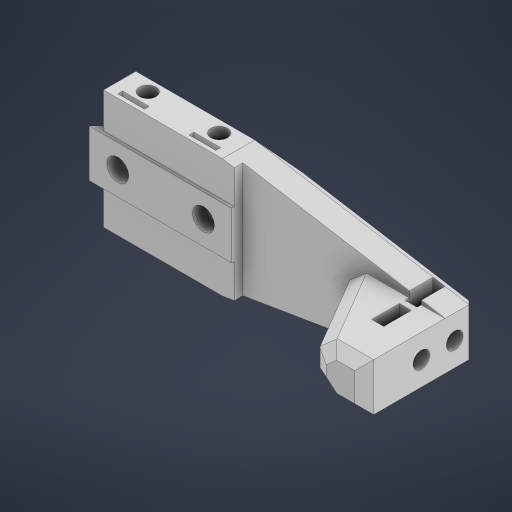
# Autodesk Inventor part: Lupfer oben
Saved by Autodesk Inventor 2024.2 (Build 282272000, 272)
## iProperties
Created: 2023-12-02
Part Number: Lupfer oben
Material: Generisch
Document SubType Name: Modeling
Designer: jacob
Density: 1 g/cm^3
Appearance: Vorgabe
Author: jacob
Autodesk Inventor part; units mm, degrees
ref_plane "YZ Plane" through (0, 0, 0) normal (1, 0, 0) x (0, 1, 0)
ref_plane "XZ Plane" through (0, 0, 0) normal (0, 1, 0) x (-1, 0, 0)
ref_plane "XY Plane" through (0, 0, 0) normal (0, 0, 1) x (1, 0, 0)
sketch "Skizze1" plane through (0, 0, 0) normal (0, 0, 1) x (1, 0, 0)
  line L0 (0, 0) -> (0, -12.5)
  line L1 (0, -12.5) -> (25, -12.5)
  line L2 (25, -12.5) -> (25, -5)
  line L3 (25, -5) -> (70, -5)
  line L4 (70, -5) -> (70, 0)
  line L5 (0, 0) -> (70, 0)
  line L6 (25, -12.5) -> (70, -5)
  dimension "d0" = 25
  dimension "d1" = 12.5
  dimension "d3" = 5
  dimension "d31" = 70
  constraints: 14 end point, 4 perpendicular, 1 horizontal, 1 horizontal alignment, 1 vertical
  measures "d0" distance of L0.end L1.end
  measures "d1" distance of L0.start L0.end
  measures "d3" distance between parallel lines of L5 L3
  measures "d31" distance of L4.end L0.start
extrude "Extrusion1" add sketch "Skizze1" along normal blind 5
sketch "Skizze2" plane through (0, 0, 5) normal (0, 0, 1) x (1, 0, 0)
  line L0 (70, 0) -> (0, 0) projected
  line L1 (0, 0) -> (0, -12.5) projected
  point P0 (3.5, 0)
  point P1 (0, 0)
  point P2 (21.5, 0)
  dimension "d7" = 3.5
  dimension "d84" = 18
  constraints: 1 horizontal alignment, 1 point on line
  measures "d7" distance of L0.end point (3.5, 0)
  measures "d84" distance of point (3.5, 0) point (21.5, 0)
hole "Bohrung1" at (3.5, 0, 5) at (21.5, 0, 5) direction (0, 0, -1) diameter 3.5 end through all
sketch "Skizze3" plane through (0, -12.5, 0) normal (0, -1, 0) x (1, 0, 0)
  line L0 (0, 0) -> (0, 5) projected
  line L1 (0, 2.5) -> (5, 2.5) construction
  line L2 (20, 2.5) -> (25, 2.5) construction
  point P0 (25, 0)
  dimension "d15" = 15
  constraints: 4 end point, 4 horizontal alignment, 3 midpoint, 2 horizontal, 1 collinear, 1 vertical alignment
  measures "d15" distance of L1.end L2.start
sketch "Skizze4" plane through (0, 0, 5) normal (0, 0, 1) x (1, 0, 0)
  line L0 (2.2, -5) -> (7.8, -5)
  line L1 (7.8, -5) -> (7.8, -7.5)
  line L2 (7.8, -7.5) -> (2.2, -7.5)
  line L3 (2.2, -7.5) -> (2.2, -5)
  line L4 (17.2, -5) -> (22.8, -5)
  line L5 (22.8, -5) -> (22.8, -7.5)
  line L6 (22.8, -7.5) -> (17.2, -7.5)
  line L7 (17.2, -7.5) -> (17.2, -5)
  line L8 (5, -5) -> (0, -5) construction
  line L9 (20, -5) -> (25, -5) construction
  line L10 (0, -12.5) -> (25, -12.5) projected
  line L11 (0, 0) -> (0, -12.5) projected
  line L12 (25, -12.5) -> (25, 0)
  line L13 (70, 0) -> (23.25, 0) projected
  dimension "d17" = 5.6
  dimension "d18" = 2.5
  dimension "d20" = 15
  dimension "d21" = 5
  constraints: 22 end point, 5 point on line, 4 parallel, 3 equal length, 3 horizontal, 3 perpendicular, 2 midpoint, 1 vertical
  measures "d17" distance of L0.start L0.end
  measures "d18" distance of L0.end L1.end
  measures "d20" distance of L9.start L8.start
  measures "d21" distance from line of L10 L5.end
extrude "Extrusion2" cut sketch "Skizze4" against normal blind 5
hole "Bohrung2" at (5, -12.5, 2.5) at (20, -12.5, 2.5) direction (0, 1, 0) diameter 3.5 depth 9 tip angle 90
mirror "Spiegeln2" about plane through (70, 0, 0) normal (0, 1, 0) of "Extrusion1", "Bohrung1", "Extrusion2", "Bohrung2"
sketch "Skizze13" plane through (0, 0, 0) normal (0, 1, 0) x (-1, 0, 0)
  line L0 (-70, 0) -> (-70, 5) projected
  line L1 (-70, 0) -> (-70, -5)
  line L2 (-70, -5) -> (0, -5)
  line L3 (0, -5) -> (0, 0)
  line L4 (0, 0) -> (-70, 0)
  dimension "d80" = 5
  dimension "d116" = 90
  constraints: 8 end point, 3 perpendicular
  measures "d80" distance of L2.end L3.end
  measures "d116" angle of L4 L1
extrude "Extrusion6" add sketch "Skizze13" along normal mid plane 10
sketch "Skizze14" plane through (21.5, 0, 0) normal (0, 0, 1) x (1, 0, 0)
  circle A0 centre (0, 0) radius 1.75 projected
  circle A1 centre (-18, 0) radius 1.75 projected
  point P0 (-21.5, 0)
  point P1 (-4, 0)
  constraints: 2 coincident
hole "Bohrung7" at (21.5, 0, 0) at (3.5, 0, 0) direction (0, 0, -1) diameter 6 end through all
sketch "Skizze15" plane through (0, 0, 0) normal (0, 1, 0) x (-1, 0, 0)
  line L0 (-70, 0) -> (-70, 5) projected
  line L1 (-70, 5) -> (-70, 22)
  line L2 (-70, 22) -> (-60, 22)
  line L3 (-60, 22) -> (-50, 5)
  line L4 (-50, 5) -> (-70, 5)
  point P0 (0, 0)
  dimension "d92" = 20
  dimension "d93" = 10
  dimension "d94" = 17
  constraints: 8 end point, 2 perpendicular, 1 vertical
  measures "d92" distance of L3.end L0.end
  measures "d93" distance of L1.end L2.end
  measures "d94" distance of L0.end L1.end
extrude "Extrusion7" add sketch "Skizze15" along normal mid plane 10
sketch "Skizze16" plane through (0, -5, 0) normal (0, -1, 0) x (1, 0, 0)
  point P0 (0, 0)
sketch "Skizze17" plane through (0, -5, 0) normal (0, -1, 0) x (1, 0, 0)
  line L0 (62.5, 0.1) -> (62.5, 5.9)
  line L1 (62.5, 5.9) -> (65, 5.9)
  line L2 (65, 5.9) -> (65, 0.1)
  line L3 (65, 7.1) -> (62.5, 7.1)
  line L4 (62.5, 7.1) -> (62.5, 12.9)
  line L5 (62.5, 12.9) -> (65, 12.9)
  line L6 (65, 12.9) -> (65, 7.1)
  line L7 (70, 5) -> (70, 22) projected
  line L8 (70, 22) -> (60, 22) construction
  line L9 (62.5, 0.1) -> (65, 0.1)
  line L10 (70, 0) -> (22.8, 0) construction
  point P0 (0, 0)
  point P1 (63.75, 5.9)
  point P2 (63.75, 7.1)
  point P3 (62.5, 10)
  point P4 (62.5, 3)
  point P5 (23, 0)
  dimension "d97" = 5.8
  dimension "d98" = 2.5
  dimension "d99" = 5
  dimension "d111" = 7
  dimension "d115" = 12
  constraints: 16 end point, 4 midpoint, 3 horizontal, 3 parallel, 2 equal length, 1 perpendicular, 1 vertical alignment
  measures "d97" distance of L0.start L0.end
  measures "d98" distance of L2.end L0.start
  measures "d99" distance between parallel lines of L7 L2
  measures "d111" distance of point (62.5, 10) point (62.5, 3)
  measures "d115" distance from line of L8 point (62.5, 10)
extrude "Extrusion8" cut sketch "Skizze17" along normal through all both and the other way through all
sketch "Skizze18" plane through (70, -5, 0) normal (1, 0, 0) x (0, 0, -1)
  line L0 (-22, 0) -> (-22, 10) construction
  line L1 (0, 10) -> (0, 0)
  line L2 (0, 6.75) -> (0, 3.25) projected
  point P0 (-10, 5)
  point P1 (-3, 5)
  point P2 (0, 5)
  point P3 (0, 5)
  dimension "d109" = 7
  dimension "d160" = 12
  constraints: 2 end point, 2 horizontal alignment, 2 midpoint, 1 vertical
  measures "d109" distance of point (-3, 5) point (-10, 5)
  measures "d160" distance from line of L0 point (-10, 5)
hole "Bohrung8" at (70, 0, 3) at (70, 0, 10) direction (-1, 0, 0) diameter 3.5 depth 12 tip angle 90
sketch "Skizze19" plane through (0, 0, 0) normal (0, 0, -1) x (-1, 0, 0)
  line L0 (-25, -12.5) -> (-70, -5) projected
  line L1 (-25, -12.5) -> (-25, -5)
  line L2 (0, -5) -> (-70, -5) projected
  line L3 (-22.8, -5) -> (-70, -5) projected
  line L4 (-25, -5) -> (-70, -5)
  line L5 (-70, -5) -> (-62.5, -6.25)
  point P0 (0, 0)
  constraints: 6 end point, 1 collinear, 1 horizontal, 1 point on line, 1 vertical
extrude "Extrusion9" add sketch "Skizze19" along normal up to surface (5 mm away)
mirror "Spiegeln3" about plane through (0, 0, 0) normal (0, 1, 0) of "Extrusion9"
chamfer "Fasen3" distance 5 angle 45 1 edges at (70, 0, -5)
chamfer "Fasen4" distance 5 angle 45 4 edges at (25, -8.75, -5) (45, -9.1667, -5) (25, 8.75, -5) (45, 9.1667, -5)
chamfer "Fasen5" distance 3 angle 45 2 edges at (55, 5, 13.5) (55, -5, 13.5)
chamfer "Fasen6" distance 2 angle 45 6 edges at (66.7403, 5, 22) (61.7403, 3.5, 22) (60, 0, 22) (61.7403, -3.5, 22) (66.7403, -5, 22) (70, 0, 22)
chamfer "Fasen7" distance 1 angle 45 2 edges at (3.5, 3, -5) (21.5, 3, -5)
chamfer "Fasen8" distance 1 angle 45 2 edges at (15, 5, -5) (14.9999, -5, -5)
chamfer "Fasen9" distance 1 angle 45 1 edges at (0, 2.9683, -5)
sketch "Skizze20" plane through (0, 0, 5) normal (0, 0, 1) x (1, 0, 0)
  circle A0 centre (3.5, 0) radius 1.75 projected
  line L0 (62.5, -6.25) -> (62.5, -5) projected
  line L1 (62.5, -5) -> (53.4805, -5) projected
  line L2 (50, -2) -> (53.4805, -5) projected
  line L3 (50, -2) -> (50, 2) projected
  line L4 (53.4805, 5) -> (50, 2) projected
  line L5 (53.4805, 5) -> (62.5, 5) projected
  line L6 (62.5, 5) -> (62.5, 6.25) projected
  line L7 (25, 12.5) -> (62.5, 6.25) projected
  line L8 (0, 12.5) -> (25, 12.5) projected
  line L9 (0, -12.5) -> (0, 12.5) projected
  line L10 (0, -12.5) -> (25, -12.5) projected
  line L11 (25, -12.5) -> (62.5, -6.25) projected
  line L12 (7.8, -5) -> (7.8, -7.5) projected
  line L13 (7.8, -7.5) -> (2.2, -7.5) projected
  line L14 (2.2, -7.5) -> (2.2, -5) projected
  line L15 (2.2, -5) -> (7.8, -5) projected
  line L16 (22.8, -5) -> (22.8, -7.5) projected
  line L17 (22.8, -7.5) -> (17.2, -7.5) projected
  line L18 (17.2, -7.5) -> (17.2, -5) projected
  line L19 (17.2, -5) -> (22.8, -5) projected
  circle A1 centre (21.5, 0) radius 1.75 projected
  circle A2 centre (3.5, 0) radius 1.75 projected
  line L20 (22.8, 7.5) -> (22.8, 5) projected
  line L21 (22.8, 5) -> (17.2, 5) projected
  line L22 (17.2, 5) -> (17.2, 7.5) projected
  line L23 (17.2, 7.5) -> (22.8, 7.5) projected
  line L24 (7.8, 7.5) -> (7.8, 5) projected
  line L25 (7.8, 5) -> (2.2, 5) projected
  line L26 (2.2, 5) -> (2.2, 7.5) projected
  line L27 (2.2, 7.5) -> (7.8, 7.5) projected
  circle A3 centre (3.5, 0) radius 2.3
  circle A4 centre (21.5, 0) radius 2.3
  line L28 (0, -12.5) -> (0, 12.5) projected
  line L29 (0, 5) -> (27.5, 5)
  line L30 (27.5, 5) -> (27.5, -5)
  line L31 (27.5, -5) -> (0, -5)
  line L32 (2.2, -5) -> (7.8, -5) projected
  line L33 (0, -5) -> (-2.5, -5)
  line L34 (-2.5, -5) -> (-2.5, 5)
  line L35 (-2.5, 5) -> (0, 5)
  line L36 (0, 5) -> (0, -5)
  point P0 (0, 0)
  point P1 (22.8, 5)
  point P2 (17.2, 5)
  point P3 (7.8, 5)
  point P4 (2.2, 5)
  point P5 (2.2, -5)
  point P6 (7.8, -5)
  point P7 (17.2, -5)
  point P8 (22.8, -5)
  dimension "d140" = 4.6
  dimension "d141" = 4.6
  dimension "d142" = 10
  dimension "d143" = 27.5
  dimension "d144" = 2.5
  constraints: 14 end point, 4 perpendicular, 2 centre point, 2 coincident, 2 parallel, 2 point on line, 1 collinear, 1 horizontal
  measures "d140" diameter of A3
  measures "d141" diameter of A4
  measures "d142" distance between parallel lines of L29 L31
  measures "d143" distance of L30.end L31.end
  measures "d144" distance of L31.end L33.end
extrude "Extrusion10" cut sketch "Skizze20" against normal blind 0.5 contours A3 | A4
extrude "Extrusion11" add sketch "Skizze20" along normal blind 2.3 contours L33 L34 L35 L9 | L9 L29 L25 L21 L30 L31 L19 L15
chamfer "Fasen10" distance 2.3 distance2 2.5 1 edges at (-2.5, 0, 5) measured on face at (-2.5, 0, 5.5)
sketch "Skizze21" plane through (0, 5, 0) normal (0, 1, 0) x (1, 0, 0)
  line L0 (2.2, -5) -> (2.2, 0) projected
  line L1 (2.2, -5) -> (2.2, -6)
  line L2 (2.2, -6) -> (7.8, -6)
  line L3 (7.8, -6) -> (7.8, -5)
  line L4 (0, -5) -> (0, -6.8)
  line L5 (0, -6.8) -> (27.5, -6.8)
  line L6 (0, -5) -> (25, -5) projected
  line L7 (27.5, -5) -> (27.5, -7.3) projected
  line L8 (27.5, -7.3) -> (-2.5, -7.3) projected
  line L9 (17.2, -5) -> (17.2, -6)
  line L10 (17.2, -6) -> (22.8, -6)
  line L11 (22.8, -6) -> (22.8, -5)
  line L12 (22.8, -5) -> (27.5, -5) projected
  point P0 (0, 0)
  dimension "d153" = 1
  dimension "d154" = 0.5
  dimension "d155" = 1
  constraints: 16 end point, 4 perpendicular, 3 vertical, 1 parallel, 1 point on line
  measures "d153" distance of L0.start L1.end
  measures "d154" distance between parallel lines of L8 L5
  measures "d155" distance of L9.start L9.end
extrude "Extrusion12" add sketch "Skizze21" along normal up to surface (7.5 mm away) contours L1 L2 L3 L6 L9 L10 L11 L12 L7 L5 L4
mirror "Spiegeln4" about plane through (0, 0, 0) normal (0, 1, 0) of "Extrusion12"
sketch "Skizze22" plane through (27.5, 12.5, 5) normal (0, 0, -1) x (-1, 0, 0)
  line L0 (2.5, 0) -> (0, -0.4167) projected
  line L1 (2.5, 0) -> (0, 0) projected
  line L2 (0, -0.4167) -> (0, 0) projected
  point P0 (27.5, -12.5)
extrude "Extrusion13" cut sketch "Skizze22" against normal up to surface (1.8 mm away)
mirror "Spiegeln5" about plane through (0, 0, 0) normal (0, 1, 0) of "Extrusion13"
